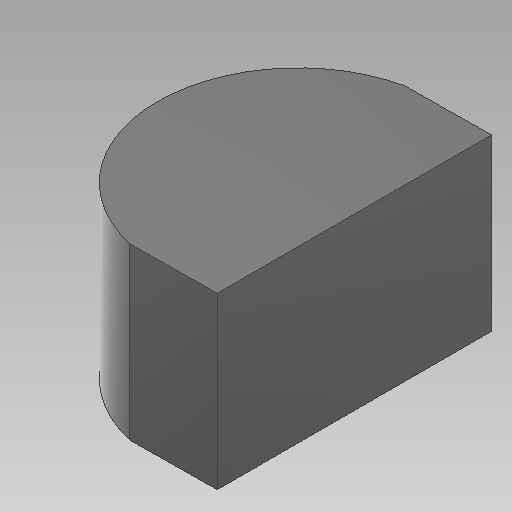
# Autodesk Inventor part: piece3
Saved by Autodesk Inventor 2020 (Build 240168000, 168)
## iProperties
Created: 2022-08-27
Part Number: piece3
Material: Acetal Resin, Black
Document SubType Name: Modeling
Designer: Umair
Density: 1.425 g/cm^3
Appearance: Smooth - Black
Author: Umair
Autodesk Inventor part; units mm, degrees
ref_plane "YZ Plane" through (0, 0, 0) normal (1, 0, 0) x (0, 1, 0)
ref_plane "XZ Plane" through (0, 0, 0) normal (0, 1, 0) x (-1, 0, 0)
ref_plane "XY Plane" through (0, 0, 0) normal (0, 0, 1) x (1, 0, 0)
sketch "Sketch1" plane through (0, 0, 0) normal (0, 1, 0) x (-1, 0, 0)
  line L0 (25, 100) -> (-25, 100)
  line L1 (-25, 100) -> (-25, -100)
  line L2 (-25, -100) -> (25, -100)
  line L3 (25, -100) -> (25, 100)
  line L4 (25, 100) -> (-25, -100) construction
  line L5 (-25, 100) -> (25, -100) construction
  point P0 (0, 0)
  dimension "d0" = 50
  dimension "d1" = 200
  constraints: 12 end point, 2 midpoint, 2 parallel, 1 horizontal, 1 perpendicular
  measures "d0" distance of L2.end L1.end
  measures "d1" distance of L1.end L0.end
extrude "Extrusion1" add sketch "Sketch1" along normal blind 62
sketch "Sketch2" plane through (-25, 0, 100) normal (0, 0, 1) x (1, 0, 0)
  line L0 (50, 62) -> (0, 62) projected
  line L1 (50, 62) -> (90, 62)
  line L2 (90, 62) -> (90, 42)
  line L3 (90, 42) -> (53.2289, 0)
  line L4 (53.2289, 0) -> (50, 0)
  line L5 (50, 62) -> (50, 0)
  point P0 (25, 0)
  dimension "d4" = 40
  dimension "d5" = 20
  dimension "d6" = 90
  constraints: 10 end point, 2 perpendicular, 1 horizontal, 1 parallel
  measures "d4" distance of L0.start L1.end
  measures "d5" distance of L1.end L2.end
  measures "d6" angle of L1 L2
extrude "Extrusion2" add sketch "Sketch2" against normal up to surface (200 mm away)
sketch "Sketch3" plane through (0, 62, 0) normal (0, 1, 0) x (1, 0, 0)
  line L0 (-25, 100) -> (-25, -100) projected
  line L1 (-25, -100) -> (-25, 100)
  line L2 (-25, 100) -> (-25, 80)
  line L3 (-25, 80) -> (-76.9615, 50)
  line L4 (-25, -100) -> (-25, -80)
  line L5 (-25, -80) -> (-76.9615, -50)
  line L6 (-76.9615, -50) -> (-76.9615, 50)
  circle A0 centre (-76.9615, 0) radius 49.9974
  circle A1 centre (-126.9564, -0.5064) radius 49.9974
  line L7 (-76.9615, -50) -> (-126.45, -50.5013)
  line L8 (-127.4628, 49.4885) -> (-76.9615, 50)
  point P0 (0, 0)
  point P1 (-76.9615, 49.9974)
  point P2 (-77.4679, 49.9949)
  point P3 (-76.9615, -1.0128)
  dimension "d9" = 20
  dimension "d10" = 60
  dimension "d11" = 120
  dimension "d12" = 20
  dimension "d13" = 60
  dimension "d14" = 120
  constraints: 16 end point, 3 point on circle, 2 point on line, 1 centre point, 1 midpoint, 1 parallel, 1 tangent, 1 vertical, 4 other
  measures "d9" distance of L0.start L2.end
  measures "d10" distance of L2.end L3.end
  measures "d11" angle of L2 L3
  measures "d12" distance of L0.end L4.end
  measures "d13" distance of L4.end L5.end
  measures "d14" angle of L5 L4
extrude "Extrusion3" add sketch "Sketch3" against normal blind 62
sketch "Sketch4" plane through (0, 62, 0) normal (0, 1, 0) x (1, 0, 0)
  line L0 (-25, -100) -> (28.2289, -100) projected
  line L1 (-25, 100) -> (-25, 80) projected
  line L2 (-25, -100) -> (-25, 100)
  line L3 (-25, 100) -> (29.4775, 197.567)
  line L4 (29.4775, 197.567) -> (135.6867, 127.811)
  line L5 (135.6867, 127.811) -> (135.6867, -104.409)
  line L6 (135.6867, -104.409) -> (110.0345, -245.7212)
  line L7 (110.0345, -245.7212) -> (-5.1754, -156.6135)
  line L8 (-5.1754, -156.6135) -> (-25, -100)
  line L9 (-76.9615, -50) -> (-76.9615, 49.9974)
  line L10 (-76.9615, 49.9974) -> (-143.8651, 145.0549)
  line L11 (-143.8651, 145.0549) -> (-248.9816, -0.0013)
  line L12 (-248.9816, -0.0013) -> (-240.1494, -166.1828)
  line L13 (-240.1494, -166.1828) -> (-110.4133, -169.4443)
  line L14 (-110.4133, -169.4443) -> (-76.9615, -50)
  line L15 (-110.4133, -169.4443) -> (-5.1754, -156.6135)
  line L16 (-143.8651, 145.0549) -> (29.4775, 197.567)
  point P0 (0, 0)
  constraints: 30 end point, 2 vertical, 1 parallel
extrude "Extrusion4" cut sketch "Sketch4" against normal blind 62 contours L3 L4 L5 L6 L7 L8 L2 L1 | L1 L2 L8 L15 L14 L9 L10 L16 L3
extrude "Extrusion5" cut sketch "Sketch4" against normal blind 62 contours L3 L4 L5 L6 L7 L8 L2 L1 | L1 L2 L8 L15 L14 L9 L10 L16 L3
sketch "Sketch5" plane through (0, 0, 0) normal (0, -1, 0) x (1, 0, 0)
  arc A0 (-77.4679, -49.9949) -> (-76.9615, -49.9974) centre (-76.9615, 0) ccw projected
  line L0 (-76.9615, -49.9974) -> (-76.9615, 49.9974)
  circle A1 centre (-76.9615, 0) radius 49.9974
  line L1 (-76.9615, 50) -> (-126.45, 50.5013) projected
  line L2 (-127.4628, -49.4885) -> (-77.4679, -49.9949) projected
  arc A2 (-108.502, 50.3195) -> (-108.502, -49.6805) centre (-97.1108, 0.3195) ccw
  line L3 (-108.502, -49.6805) -> (-108.502, 50.3195) construction
  line L4 (-108.502, -49.6805) -> (-8.502, -49.6805) construction
  line L5 (-108.502, -49.6805) -> (-108.502, 50.3195)
  arc A3 (-108.502, 50.3195) -> (-108.502, -49.6805) centre (-131.0507, 0.3195) ccw
  point P0 (0, 0)
  dimension "d21" = 90
  constraints: 8 end point, 4 point on circle, 3 centre point, 2 point on line, 1 coincident, 1 horizontal, 1 perpendicular, 1 vertical
  measures "d21" angle of L4 L3
extrude "Extrusion6" cut sketch "Sketch5" against normal blind 62 contours A3 A2
body "Solid1"
